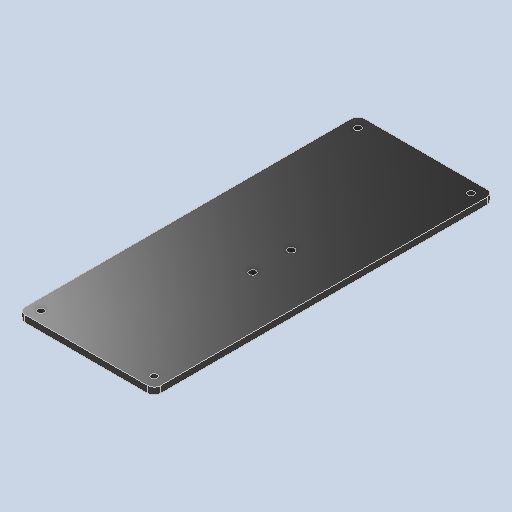
# Autodesk Inventor part: MatTren
Saved by Autodesk Inventor 2023 (Build 270158000, 158)
## iProperties
Created: 2023-10-20
Part Number: MatTren
Material: Generic
Document SubType Name: Modeling
Designer: Admins
Density: 1 g/cm^3
Appearance: Glossy - Black
Author: Admins
Autodesk Inventor part; units mm, degrees
ref_plane "YZ Plane" through (0, 0, 0) normal (1, 0, 0) x (0, 1, 0)
ref_plane "XZ Plane" through (0, 0, 0) normal (0, 1, 0) x (-1, 0, 0)
ref_plane "XY Plane" through (0, 0, 0) normal (0, 0, 1) x (1, 0, 0)
sketch "Sketch1" plane through (0, 0, 0) normal (0, 1, 0) x (-1, 0, 0)
  line L0 (-30, 75) -> (30, 75)
  line L1 (30, 75) -> (30, -75)
  line L2 (30, -75) -> (-30, -75)
  line L3 (-30, -75) -> (-30, 75)
  line L4 (30, 75) -> (25, 75)
  line L5 (25, 75) -> (25, 70)
  line L6 (25, 70) -> (30, 70)
  line L7 (30, 70) -> (30, 75)
  line L8 (-30, 75) -> (-25, 75)
  line L9 (-25, 75) -> (-25, 70)
  line L10 (-25, 70) -> (-30, 70)
  line L11 (-30, 70) -> (-30, 75)
  line L12 (30, -75) -> (25, -75)
  line L13 (25, -75) -> (25, -70)
  line L14 (25, -70) -> (30, -70)
  line L15 (30, -70) -> (30, -75)
  line L16 (-30, -75) -> (-25, -75)
  line L17 (-25, -75) -> (-25, -70)
  line L18 (-25, -70) -> (-30, -70)
  line L19 (-30, -70) -> (-30, -75)
  circle A0 centre (25, 70) radius 1.4
  circle A1 centre (-25, 70) radius 1.4
  circle A2 centre (25, -70) radius 1.4
  circle A3 centre (-25, -70) radius 1.4
  line L20 (-9.515, 11.025) -> (9.515, 11.025)
  line L21 (9.515, 11.025) -> (9.515, -11.025)
  line L22 (9.515, -11.025) -> (-9.515, -11.025)
  line L23 (-9.515, -11.025) -> (-9.515, 11.025)
  line L24 (-9.515, 11.025) -> (9.515, -11.025) construction
  line L25 (9.515, 11.025) -> (-9.515, -11.025) construction
  line L26 (-9.515, -11.025) -> (-7.015, -11.025)
  line L27 (-7.015, -11.025) -> (-7.015, -8.525)
  line L28 (-7.015, -8.525) -> (-9.515, -8.525)
  line L29 (-9.515, -8.525) -> (-9.515, -11.025)
  line L30 (-9.515, 11.025) -> (-7.015, 11.025)
  line L31 (-7.015, 11.025) -> (-7.015, 8.525)
  line L32 (-7.015, 8.525) -> (-9.515, 8.525)
  line L33 (-9.515, 8.525) -> (-9.515, 11.025)
  circle A4 centre (-7.015, 8.525) radius 1.5
  circle A5 centre (-7.015, -8.525) radius 1.5
  line L34 (9.515, 0) -> (8.515, 0)
  line L35 (6.515, -11.025) -> (10.515, -11.025)
  line L36 (10.515, -11.025) -> (10.515, 11.025)
  line L37 (10.515, 11.025) -> (6.515, 11.025)
  line L38 (6.515, 11.025) -> (6.515, -11.025)
  line L39 (6.515, -11.025) -> (10.515, 11.025) construction
  line L40 (10.515, -11.025) -> (6.515, 11.025) construction
  line L41 (0, -75) -> (-20, -75)
  line L42 (0, -75) -> (20, -75)
  point P0 (0, 0)
  point P1 (0, 0)
  dimension "d0" = 60
  dimension "d1" = 150
  dimension "d2" = 5
  dimension "d3" = 5
  dimension "d4" = 5
  dimension "d5" = 5
  dimension "d6" = 5
  dimension "d8" = 5
  dimension "d10" = 2.8
  dimension "d11" = 2.8
  dimension "d12" = 19.03
  dimension "d13" = 22.05
  dimension "d14" = 2.5
  dimension "d15" = 2.5
  dimension "d16" = 2.5
  dimension "d17" = 2.5
  dimension "d18" = 3
  dimension "d19" = 3
  dimension "d20" = 1
  dimension "d21" = 4
  constraints: 86 end point, 18 parallel, 12 horizontal, 9 perpendicular, 6 centre point, 6 coincident, 6 midpoint
  measures "d0" distance of L2.start L19.end
  measures "d1" distance of L1.start L2.start
  measures "d2" distance of L6.end L5.end
  measures "d3" distance of L5.end L4.end
  measures "d4" distance of L9.end L10.end
  measures "d5" distance of L8.end L9.end
  measures "d6" distance of L13.end L14.end
  measures "d8" distance of L18.end L18.start
  measures "d10" diameter of A0
  measures "d11" diameter of A1
  measures "d12" distance of L22.start L23.start
  measures "d13" distance of L20.end L22.start
  measures "d14" distance of L28.end L28.start
  measures "d15" distance of L28.start L27.start
  measures "d16" distance of L31.end L32.end
  measures "d17" distance of L31.start L31.end
  measures "d18" diameter of A4
  measures "d19" diameter of A5
  measures "d20" distance of L34.start L34.end
  measures "d21" distance of L37.end L37.start
extrude "Extrusion1" add sketch "Sketch1" along normal blind 3 contours L0 L9 A1 L10 L3 | L0 L5 A0 L6 L1 L14 A2 L13 L2 L17 A3 L18 L3 L10 A1 L9 | L0 L1 L6 A0 L5 | L18 A3 L17 L2 L3 | L1 L2 L13 A2 L14 | L20 L31 A4 L32 L23 | L20 L38 L22 L27 A5 L28 L23 L32 A4 L31 | L20 L21 L22 L38 | L28 A5 L27 L22 L23 | L37 L36 L35 L21
fillet "Fillet1" radius 2.8 1 edges at (30, 1.5, 75)
fillet "Fillet2" radius 2.8 1 edges at (-30, 1.5, 75)
fillet "Fillet3" radius 2.8 1 edges at (-30, 1.5, -75)
fillet "Fillet4" radius 2.8 1 edges at (30, 1.5, -75)
body "Solid1"
